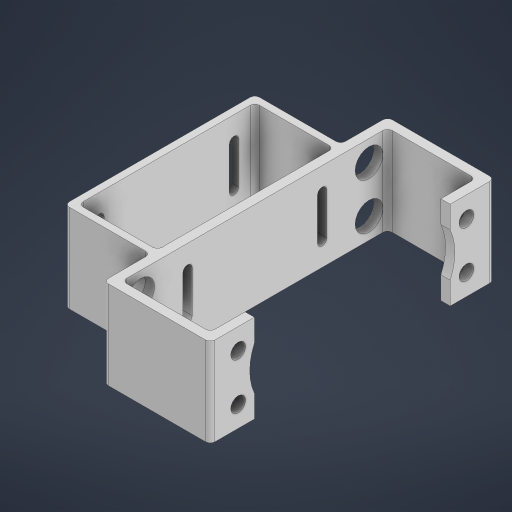
# Autodesk Inventor part: soporte_camara
Saved by Autodesk Inventor 2023.1 (Build 271208000, 208)
## iProperties
Created: 2022-11-24
Part Number: soporte_camara
Material: Generic
Document SubType Name: Modeling
Designer: amtat
Density: 1 g/cm^3
Appearance: Default
Author: amtat
Autodesk Inventor part; units mm, degrees
ref_plane "YZ Plane" through (0, 0, 0) normal (1, 0, 0) x (0, 1, 0)
ref_plane "XZ Plane" through (0, 0, 0) normal (0, 1, 0) x (-1, 0, 0)
ref_plane "XY Plane" through (0, 0, 0) normal (0, 0, 1) x (1, 0, 0)
sketch "Sketch1" plane through (0, 0, 0) normal (1, 0, 0) x (0, 1, 0)
  circle A0 centre (0, 0) radius 1.6
  line L0 (0, 0) -> (10, 0)
  circle A1 centre (10, 0) radius 1.6
  line L1 (10, 0) -> (10, -49.2)
  line L2 (10, 0) -> (59.2, 0) construction
  line L3 (10, -49.2) -> (0, -49.2)
  circle A2 centre (10, -49.2) radius 1.6
  circle A3 centre (0, -49.2) radius 1.6
  line L4 (0, -49.2) -> (0, -53.2)
  line L5 (0, -53.2) -> (15, -53.2)
  line L6 (15, -53.2) -> (15, -45.2)
  line L7 (15, -45.2) -> (-5, -45.2)
  line L8 (-5, -45.2) -> (-5, -53.2)
  line L9 (-5, -53.2) -> (0, -53.2)
  line L10 (0, 0) -> (0, -24.6)
  line L11 (0, -24.6) -> (3.1237, -24.6)
  line L12 (0, 4) -> (15, 4)
  line L13 (15, 4) -> (15, -4)
  line L14 (15, -4) -> (-5, -4)
  line L15 (-5, -4) -> (-5, 4)
  line L16 (-5, 4) -> (0, 4)
  dimension "d0" = 3.2
  dimension "d1" = 10
  dimension "d2" = 3.2
  dimension "d3" = 49.2
  dimension "d4" = 90
  dimension "d5" = 3.2
  dimension "d6" = 3.2
  dimension "d7" = 4
  dimension "d8" = 15
  dimension "d9" = 8
  dimension "d10" = 90
  dimension "d11" = 20
  dimension "d12" = 24.6
  constraints: 34 end point, 6 perpendicular, 5 symmetric about line, 4 centre point, 4 coincident, 4 horizontal, 3 vertical
  measures "d0" diameter of A0
  measures "d1" distance of L0.start L0.end
  measures "d2" diameter of A1
  measures "d3" distance of L1.start L1.end
  measures "d4" angle of L1 L2
  measures "d5" diameter of A2
  measures "d6" diameter of A3
  measures "d7" distance of L4.start L4.end
  measures "d8" distance of L4.end L5.end
  measures "d9" distance of L5.end L6.end
  measures "d10" angle of L6 L5
  measures "d11" distance of L6.end L7.end
  measures "d12" distance of L0.start L10.end
extrude "Extrusion1" add sketch "Sketch1" along normal blind 2 contours L0 A1 L1 L14 L10 A0 | A0 L10 L14 L15 L16 L12 L13 L1 A1 L0 | L7 L6 L5 L4 A3 L3 A2 L1 | L1 A2 L3 A3 L4 L9 L8 L7
sketch "Sketch2" plane through (2, 0, 0) normal (1, 0, 0) x (0, 0, -1)
  line L0 (4, 15) -> (-4, 15) projected
  line L1 (-4, 15) -> (-4, -5) projected
  line L2 (-4, -5) -> (4, -5) projected
  line L3 (4, -5) -> (4, 15) projected
  circle A0 centre (0, 10) radius 1.6 projected
  circle A1 centre (0, 0) radius 1.6 projected
  line L4 (53.2, 15) -> (45.2, 15) projected
  line L5 (45.2, 15) -> (45.2, -5) projected
  line L6 (45.2, -5) -> (53.2, -5) projected
  line L7 (53.2, -5) -> (53.2, 15) projected
  circle A2 centre (49.2, 0) radius 1.6 projected
  circle A3 centre (49.2, 10) radius 1.6 projected
  line L8 (4, -5) -> (4, 15) projected
  line L9 (4, 15) -> (4, 5)
  line L10 (4, 5) -> (14, 5)
  arc A4 (4, 10.6789) -> (4, -0.6789) centre (14, 5) ccw
  line L11 (0, 0) -> (24.6, 0)
  line L12 (24.6, 0) -> (24.6, 10.6789)
  arc A5 (45.2, -0.6789) -> (45.2, 10.6789) centre (35.2, 5) ccw
  point P0 (45.2, -0.6789)
  point P1 (3.6438, 0)
  point P2 (4, 0)
  point P3 (4, 10.6789)
  dimension "d15" = 10
  dimension "d16" = 10
  dimension "d17" = 23
  dimension "d18" = 24.6
  constraints: 8 end point, 4 point on circle, 3 symmetric about line, 2 centre point, 2 perpendicular, 2 point on line, 1 coincident, 1 horizontal, 1 midpoint, 1 other
  measures "d15" distance of L0.start L9.end
  measures "d16" distance of L9.end L10.end
  measures "d17" diameter of A4
  measures "d18" distance of L11.start L11.end
extrude "Extrusion2" cut sketch "Sketch2" against normal blind 2 contours L3 L11 A4 | A5 L5 picked at (3.5828, 2.5409)
sketch "Sketch3" plane through (2, 0, 0) normal (1, 0, 0) x (0, 0, -1)
  arc A0 (4, 10.6789) -> (3.6438, 0) centre (14, 5) ccw projected
  line L0 (4, 10.6789) -> (4, 15) projected
  line L1 (4, 15) -> (-4, 15) projected
  line L2 (-4, 15) -> (-4, -5) projected
  line L3 (-4, -5) -> (4, -5) projected
  line L4 (4, -5) -> (4, 0) projected
  line L5 (4, 0) -> (3.6438, 0) projected
  circle A1 centre (0, 10) radius 1.6 projected
  circle A2 centre (0, 0) radius 1.6 projected
  arc A3 (45.2, -0.6789) -> (45.2, 10.6789) centre (35.2, 5) ccw projected
  line L6 (45.2, -0.6789) -> (45.2, -5) projected
  line L7 (45.2, -5) -> (53.2, -5) projected
  line L8 (53.2, -5) -> (53.2, 15) projected
  line L9 (53.2, 15) -> (45.2, 15) projected
  line L10 (45.2, 15) -> (45.2, 10.6789) projected
  circle A4 centre (49.2, 0) radius 1.6 projected
  circle A5 centre (49.2, 10) radius 1.6 projected
  line L11 (-4, -5) -> (4, -5) projected
  line L12 (-4, -5) -> (-6, -5)
  line L13 (-6, -5) -> (-6, 15)
  line L14 (-6, 15) -> (-4, 15)
  line L15 (53.2, 15) -> (45.2, 15) projected
  line L16 (53.2, 15) -> (55.2, 15)
  line L17 (55.2, 15) -> (55.2, -5)
  line L18 (55.2, -5) -> (53.2, -5)
  dimension "d21" = 2
  dimension "d22" = 2
  constraints: 12 end point, 4 perpendicular, 2 horizontal
  measures "d21" distance of L2.end L12.end
  measures "d22" distance of L8.end L16.end
extrude "Extrusion3" add sketch "Sketch3" against normal blind 20 contours L2 L12 L13 L14 | L8 L16 L17 L18
sketch "Sketch4" plane through (0, 15, -45.2) normal (0, 1, 0) x (1, 0, 0)
  line L0 (0, -41.2) -> (0, -49.2) projected
  line L1 (0, -49.2) -> (-18, -49.2) projected
  line L2 (-18, -51.2) -> (-18, -49.2) projected
  line L3 (2, -51.2) -> (-18, -51.2) projected
  line L4 (2, -41.2) -> (2, -51.2) projected
  line L5 (0, -41.2) -> (2, -41.2) projected
  line L6 (0, 8) -> (0, 0) projected
  line L7 (0, 0) -> (2, 0) projected
  line L8 (2, 10) -> (2, 0) projected
  line L9 (2, 10) -> (-18, 10) projected
  line L10 (-18, 8) -> (-18, 10) projected
  line L11 (0, 8) -> (-18, 8) projected
  point P0 (0, -45.2)
extrude "Extrusion4" cut sketch "Sketch4" against normal blind 0.5
sketch "Sketch5" plane through (0, -5, -4) normal (0, -1, 0) x (1, 0, 0)
  line L0 (0, 8) -> (0, 0) projected
  line L1 (0, 0) -> (2, 0) projected
  line L2 (2, 10) -> (2, 0) projected
  line L3 (2, 10) -> (-18, 10) projected
  line L4 (-18, 8) -> (-18, 10) projected
  line L5 (0, 8) -> (-18, 8) projected
  line L6 (0, -41.2) -> (0, -49.2) projected
  line L7 (0, -49.2) -> (-18, -49.2) projected
  line L8 (-18, -51.2) -> (-18, -49.2) projected
  line L9 (2, -51.2) -> (-18, -51.2) projected
  line L10 (2, -41.2) -> (2, -51.2) projected
  line L11 (0, -41.2) -> (2, -41.2) projected
  point P0 (0, 4)
extrude "Extrusion5" cut sketch "Sketch5" against normal blind 0.5
sketch "Sketch6" plane through (0, 0, 0) normal (-1, 0, 0) x (0, 0, 1)
  circle A0 centre (-49.2, 10) radius 1.6 projected
  circle A1 centre (-49.2, 0) radius 1.6 projected
  line L0 (-53.2, -4.5) -> (-45.2, -4.5) projected
  line L1 (-45.2, -0.6789) -> (-45.2, -4.5) projected
  arc A2 (-45.2, 10.6789) -> (-45.2, -0.6789) centre (-35.2, 5) ccw projected
  line L2 (-45.2, 14.5) -> (-45.2, 10.6789) projected
  line L3 (-45.2, 14.5) -> (-53.2, 14.5) projected
  line L4 (-53.2, -4.5) -> (-53.2, 14.5) projected
  circle A3 centre (0, 0) radius 1.6 projected
  circle A4 centre (0, 10) radius 1.6 projected
  line L5 (-4, -4.5) -> (4, -4.5) projected
  line L6 (4, 14.5) -> (4, -4.5) projected
  line L7 (4, 14.5) -> (-4, 14.5) projected
  line L8 (-4, 10.6789) -> (-4, 14.5) projected
  arc A5 (-3.6438, 0) -> (-4, 10.6789) centre (-14, 5) ccw projected
  line L9 (-3.6438, 0) -> (-4, 0) projected
  line L10 (-4, -4.5) -> (-4, 0) projected
  line L11 (-45.2, 14.5) -> (-45.2, 10.6789) projected
  line L12 (-45.2, 14.5) -> (-45.7, 14.5)
  line L13 (-45.2, 14.5) -> (-53.2, 14.5) projected
  line L14 (-45.7, 14.5) -> (-45.7, -4.5)
  line L15 (-45.2, -4.5) -> (-55.2, -4.5) projected
  line L16 (-4, -4.5) -> (-4, 0) projected
  line L17 (-4, -4.5) -> (-3.5, -4.5)
  line L18 (-3.5, -4.5) -> (-3.5, 14.5)
  line L19 (4, 14.5) -> (-4, 14.5) projected
  point P0 (-3.5, 0.3096)
  point P1 (-3.5, 9.6904)
  point P2 (-45.7, 0.3096)
  point P3 (-45.7, 9.6904)
  dimension "d29" = 0.5
  dimension "d30" = 0.5
  constraints: 8 end point, 4 point on line, 2 perpendicular
  measures "d29" distance of L2.start L12.end
  measures "d30" distance of L5.start L17.end
extrude "Extrusion6" cut sketch "Sketch6" against normal through all contours L14 A2 L1 L0 | L3 L2 A2 L14 | L10 L9 A5 L18 L5 | A5 L8 L7 L18
sketch "Sketch7" plane through (-18, 0, 0) normal (-1, 0, 0) x (0, 0, 1)
  line L0 (-55.2, -4.5) -> (-53.2, -4.5) projected
  line L1 (-53.2, -4.5) -> (-53.2, 14.5) projected
  line L2 (-53.2, 14.5) -> (-55.2, 14.5) projected
  line L3 (-55.2, 14.5) -> (-55.2, -4.5) projected
  line L4 (4, 14.5) -> (4, -4.5) projected
  line L5 (4, -4.5) -> (6, -4.5) projected
  line L6 (6, -4.5) -> (6, 14.5) projected
  line L7 (6, 14.5) -> (4, 14.5) projected
  line L8 (4, 14.5) -> (4, -4.5) projected
  line L9 (-55.2, 14.5) -> (-45.7, 14.5) projected
  line L10 (-3.5, 14.5) -> (6, 14.5) projected
  line L11 (-55.2, 14.5) -> (6, 14.5)
  line L12 (-45.7, -4.5) -> (-55.2, -4.5) projected
  line L13 (6, -4.5) -> (-3.5, -4.5) projected
  line L14 (-55.2, -4.5) -> (6, -4.5)
  point P0 (0, 0)
  point P1 (-3.5, -4.5)
  constraints: 4 end point, 2 horizontal
extrude "Extrusion7" add sketch "Sketch7" along normal blind 2
sketch "Sketch8" plane through (-20, 0, 0) normal (-1, 0, 0) x (0, 0, 1)
  circle A0 centre (0, 10) radius 1.6 projected
  circle A1 centre (0, 0) radius 1.6 projected
  circle A2 centre (-49.2, 10) radius 1.6 projected
  circle A3 centre (-49.2, 0) radius 1.6 projected
  circle A4 centre (-49.2, 10) radius 3
  circle A5 centre (-49.2, 0) radius 3
  circle A6 centre (0, 0) radius 3
  circle A7 centre (0, 10) radius 3
  dimension "d35" = 6
  dimension "d36" = 6
  dimension "d37" = 6
  dimension "d38" = 6
  constraints: 4 centre point, 4 coincident
  measures "d35" diameter of A4
  measures "d36" diameter of A5
  measures "d37" diameter of A6
  measures "d38" diameter of A7
extrude "Extrusion8" cut sketch "Sketch8" against normal blind 2 contours A0 | A1 | A2 | A3 | A4 | A5 | A6 | A7
sketch "Sketch9" plane through (-20, 0, 0) normal (-1, 0, 0) x (0, 0, 1)
  circle A0 centre (0, 0) radius 3 projected
  circle A1 centre (-49.2, 0) radius 3 projected
  circle A2 centre (0, 10) radius 3 projected
  circle A3 centre (-49.2, 10) radius 3 projected
  line L0 (-55.2, -4.5) -> (6, -4.5) projected
  line L1 (6, -4.5) -> (6, 14.5) projected
  line L2 (6, 14.5) -> (-55.2, 14.5) projected
  line L3 (-55.2, 14.5) -> (-55.2, -4.5) projected
extrude "Extrusion9" add sketch "Sketch9" along normal blind 1
sketch "Sketch10" plane through (-18, 0, 0) normal (1, 0, 0) x (0, 0, -1)
  circle A0 centre (0, 0) radius 3 projected
  circle A1 centre (49.2, 0) radius 3 projected
  circle A2 centre (0, 10) radius 3 projected
  circle A3 centre (49.2, 10) radius 3 projected
  line L0 (-4, 14.5) -> (-4, -4.5) projected
  line L1 (53.2, -4.5) -> (-4, -4.5) projected
  line L2 (53.2, -4.5) -> (53.2, 14.5) projected
  line L3 (-4, 14.5) -> (53.2, 14.5) projected
extrude "Extrusion10" cut sketch "Sketch10" against normal blind 1
sketch "Sketch11" plane through (-21, 0, 0) normal (-1, 0, 0) x (0, 0, 1)
  line L0 (6, -4.5) -> (6, 14.5) projected
  line L1 (6, 14.5) -> (-55.2, 14.5) projected
  line L2 (-55.2, 14.5) -> (-55.2, -4.5) projected
  line L3 (-55.2, -4.5) -> (6, -4.5) projected
  circle A0 centre (0, 0) radius 3 projected
  circle A1 centre (-49.2, 0) radius 3 projected
  circle A2 centre (0, 10) radius 3 projected
  circle A3 centre (-49.2, 10) radius 3 projected
  line L4 (6, -4.5) -> (-3.5, -4.5) projected
  line L5 (6, -4.5) -> (-24.6, -4.5)
  line L6 (-24.6, -4.5) -> (-43.6, -4.5)
  line L7 (-55.2, -4.5) -> (6, -4.5) projected
  line L8 (-43.6, -4.5) -> (-45.1, -4.5)
  line L9 (-43.6, -4.5) -> (-42.1, -4.5) construction
  line L10 (-45.1, -4.5) -> (-45.1, 14.5)
  line L11 (6, 14.5) -> (-55.2, 14.5) projected
  line L12 (-45.1, 14.5) -> (-43.6, 14.5)
  line L13 (-43.6, 14.5) -> (-43.6, -4.5)
  line L14 (-24.6, -4.5) -> (-5.6, -4.5)
  line L15 (-24.6, -4.5) -> (-5.6, -4.5) construction
  line L16 (-5.6, -4.5) -> (-4.1, -4.5)
  line L17 (-4.1, -4.5) -> (-4.1, 14.5)
  line L18 (-4.1, 14.5) -> (-5.6, 14.5)
  line L19 (-5.6, 14.5) -> (-5.6, -4.5)
  dimension "d45" = 30.6
  dimension "d46" = 19
  dimension "d47" = 1.5
  dimension "d48" = 180
  dimension "d49" = 1.5
  dimension "d50" = 19
  dimension "d51" = 0
  dimension "d52" = 1.5
  dimension "d53" = 1.5
  constraints: 26 end point, 6 point on line, 4 collinear, 2 horizontal, 2 perpendicular, 1 midpoint
  measures "d45" distance of L0.start L5.end
  measures "d46" distance of L5.end L6.end
  measures "d47" distance of L6.end L8.end
  measures "d48" angle of L8 L9
  measures "d49" distance of L10.end L12.end
  measures "d50" distance of L5.end L14.end
  measures "d51" distance between parallel lines of L14 L15
  measures "d52" distance of L14.end L16.end
  measures "d53" distance of L17.end L18.end
extrude "Extrusion11" add sketch "Sketch11" along normal blind 17 contours L17 L3 L19 L1 | L13 L3 L10 L1
sketch "Sketch12" plane through (-38, 0, 0) normal (-1, 0, 0) x (0, 0, 1)
  line L0 (-5.6, -4.5) -> (-4.1, -4.5) projected
  line L1 (-4.1, -4.5) -> (-4.1, 14.5) projected
  line L2 (-4.1, 14.5) -> (-5.6, 14.5) projected
  line L3 (-5.6, 14.5) -> (-5.6, -4.5) projected
  line L4 (-43.6, 14.5) -> (-45.1, 14.5) projected
  line L5 (-45.1, 14.5) -> (-45.1, -4.5) projected
  line L6 (-45.1, -4.5) -> (-43.6, -4.5) projected
  line L7 (-43.6, -4.5) -> (-43.6, 14.5) projected
  line L8 (-43.6, -4.5) -> (-5.6, -4.5) projected
  line L9 (-5.6, 14.5) -> (-43.6, 14.5) projected
  point P0 (0, 0)
extrude "Extrusion12" add sketch "Sketch12" along normal blind 1.5
sketch "Sketch13" plane through (-39.5, 0, 0) normal (-1, 0, 0) x (0, 0, 1)
  line L0 (-4.1, 14.5) -> (-45.1, 14.5) projected
  line L1 (-45.1, 14.5) -> (-45.1, -4.5) projected
  line L2 (-45.1, -4.5) -> (-4.1, -4.5) projected
  line L3 (-4.1, -4.5) -> (-4.1, 14.5) projected
  line L4 (-45.1, -4.5) -> (-4.1, -4.5) projected
  line L5 (-45.1, -4.5) -> (-40.1, -4.5)
  line L6 (-40.1, -4.5) -> (-40.1, -0.5)
  line L7 (-43.6, -4.5) -> (-5.6, -4.5) projected
  line L8 (-40.1, -4.5) -> (-36.1, -4.5) construction
  line L9 (-40.1, -0.5) -> (-38.1, -0.5)
  line L10 (-38.1, -0.5) -> (-38.1, 10.5)
  line L11 (-38.1, 10.5) -> (-40.1, 10.5)
  line L12 (-40.1, 10.5) -> (-40.1, -0.5)
  line L13 (-45.1, -4.5) -> (-24.6, -4.5)
  line L14 (-24.6, -4.5) -> (-24.6, 1.3514)
  line L15 (-9.1, -0.5) -> (-11.1, -0.5)
  line L16 (-11.1, -0.5) -> (-11.1, 10.5)
  line L17 (-11.1, 10.5) -> (-9.1, 10.5)
  line L18 (-9.1, 10.5) -> (-9.1, -0.5)
  point P0 (0, 0)
  dimension "d58" = 5
  dimension "d59" = 4
  dimension "d60" = 270
  dimension "d61" = 2
  dimension "d62" = 11
  dimension "d63" = 2
  dimension "d64" = 20.5
  constraints: 26 end point, 5 perpendicular, 4 symmetric about line, 2 point on line, 1 horizontal, 1 midpoint
  measures "d58" distance of L1.end L5.end
  measures "d59" distance of L5.end L6.end
  measures "d61" distance of L6.end L9.end
  measures "d62" distance of L9.end L10.end
  measures "d63" distance of L10.end L11.end
  measures "d64" distance of L1.end L13.end
extrude "Extrusion13" cut sketch "Sketch13" against normal through all contours L12 L11 L10 L9 | L15 L16 L17 L18
fillet "Fillet1" radius 1 16 edges at (-38.75, 10.5, -40.1) (-38.75, 10.5, -38.1) (-38.75, 10.5, -11.1) (-38.75, 10.5, -9.1) (-38.75, -0.5, -9.1) (-38.75, -0.5, -11.1) (-38.75, -0.5, -38.1) (-38.75, -0.5, -40.1) (-20, 10.5, -40.1) (-20, 10.5, -38.1) (-20, -0.5, -38.1) (-20, -0.5, -40.1) (-20, -0.5, -11.1) (-20, -0.5, -9.1) (-20, 10.5, -9.1) (-20, 10.5, -11.1)
fillet "Fillet2" radius 1 12 edges at (-21, 5, -4.1) (-21, 5, 6) (-21, 5, -45.1) (-21, 5, -55.2) (-21, 5, -5.6) (-21, 5, -43.6) (-39.5, 5, -4.1) (-39.5, 5, -45.1) (-38, 5, -43.6) (-38, 5, -5.6) (2, 5, 6) (2, 5, -55.2)
fillet "Fillet3" radius 1 2 edges at (-19, 5, -53.2) (-19, 5, 4)
fillet "Fillet4" radius 1 2 edges at (0, 5, 4) (0, 5, -53.2)
body "Solid1"
